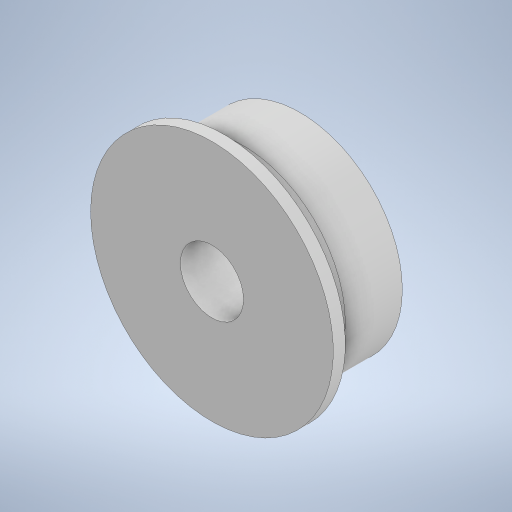
# Autodesk Inventor part: Crankshaft Bearing
Saved by Autodesk Inventor 2023 (Build 270158000, 158)
## iProperties
Created: 2023-02-24
Part Number: Crankshaft Bearing
Material: Generic
Document SubType Name: Modeling
Designer: tommy
Density: 1 g/cm^3
Appearance: Default
Author: tommy
Autodesk Inventor part; units mm, degrees
ref_plane "YZ Plane" through (0, 0, 0) normal (1, 0, 0) x (0, 1, 0)
ref_plane "XZ Plane" through (0, 0, 0) normal (0, 1, 0) x (-1, 0, 0)
ref_plane "XY Plane" through (0, 0, 0) normal (0, 0, 1) x (1, 0, 0)
sketch "Sketch1" plane through (0, 0, 0) normal (0, 1, 0) x (-1, 0, 0)
  line L0 (3.81, 0) -> (7.62, 0)
  line L1 (7.62, 0) -> (7.62, -0.3789)
  line L2 (3.81, 0) -> (3.81, -0.3789)
  line L3 (3.81, -0.3789) -> (3.81, -2.7665)
  line L4 (4.8022, -2.7665) -> (4.8022, 0)
  arc A0 (7.62, -0.3789) -> (7.0231, -0.9758) centre (7.62, -0.9758) ccw
  line L5 (7.0231, -0.9758) -> (7.0231, -2.7665)
  line L6 (7.0231, -2.7665) -> (3.81, -2.7665)
  point P0 (0, 0)
  constraints: 14 end point, 2 point on circle, 2 point on line, 1 centre point, 1 horizontal, 1 perpendicular, 1 vertical
revolve "Revolution1" add sketch "Sketch1" angle 360 about axis through (-3.81, 0, -0.3789) along (0, 0, -1) contours L0 L1 A0 L5 L6 L4
body "Solid1"
